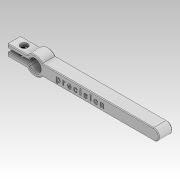
# Autodesk Inventor part: TestLever
Saved by Autodesk Inventor 2020 (Build 240168000, 168)
## iProperties
Created: 2022-01-15
Part Number: TestLever
Material: Generic
Document SubType Name: Modeling
Designer: DDeGo
Density: 1 g/cm^3
Appearance: Default
Author: DDeGo
Autodesk Inventor part; units mm, degrees
ref_plane "YZ Plane" through (0, 0, 0) normal (1, 0, 0) x (0, 1, 0)
ref_plane "XZ Plane" through (0, 0, 0) normal (0, 1, 0) x (-1, 0, 0)
ref_plane "XY Plane" through (0, 0, 0) normal (0, 0, 1) x (1, 0, 0)
sketch "Sketch1" plane through (0, 0, 0) normal (0, 0, 1) x (1, 0, 0)
  line L0 (-32.5361, 0) -> (32.5361, 0) construction
  line L1 (-32.5361, -2.5) -> (32.5361, -2.5)
  line L2 (32.5361, 2.5) -> (-32.5361, 2.5)
  arc A0 (-32.5361, 2.5) -> (-32.5361, -2.5) centre (-32.5361, 0) ccw construction
  arc A1 (32.5361, -2.5) -> (32.5361, 2.5) centre (32.5361, 0) ccw
  circle A2 centre (-20.4639, 0) radius 2.65
  arc A3 (-24.5361, -0.8) -> (-24.5361, 0.8) centre (-20.4639, 0) ccw
  line L3 (-32.5361, 2.5) -> (-32.5361, 0.8)
  line L4 (-32.5361, 0.8) -> (-24.5361, 0.8)
  line L5 (-32.5361, -2.5) -> (-32.5361, -0.8)
  line L6 (-32.5361, -0.8) -> (-24.5361, -0.8)
  line L7 (-24.5361, 0.8) -> (-22.9903, 0.8)
  line L8 (-24.5361, -0.8) -> (-22.9903, -0.8)
  point P0 (0, 0)
  point P1 (-17.1514, 2.5)
  point P2 (-23.7764, 2.5)
  point P3 (-23.7764, -2.5)
  point P4 (-17.1514, -2.5)
  dimension "d0" = 5
  dimension "d2" = 1.7
  dimension "d3" = 8
  dimension "d4" = 5.3
  dimension "d5" = 1.5
  dimension "d11" = 1.6
  dimension "d24" = 53
  constraints: 20 end point, 8 point on circle, 4 centre point, 4 tangent, 3 point on line, 2 parallel, 2 perpendicular, 1 coincident, 1 collinear, 1 horizontal, 1 midpoint, 1 vertical
  measures "d0" distance between parallel lines of L1 L2
  measures "d2" distance of L2.end L3.end
  measures "d3" distance of L3.end L4.end
  measures "d4" diameter of A2
  measures "d5" radial gap between concentric circles of A2 A3
  measures "d11" distance between parallel lines of L6 L4
  measures "d24" distance of L0.end A2.centre
extrude "Extrusion1" add sketch "Sketch1" along normal mid plane 6 contours L5 L6 A3 L1 | A3 L8 A2 L1 | L1 A2 A3 | A3 L2 A1 L1 | L1 A2 L2 A3 | L2 A2 A3 | L7 A3 L2 A2 | A3 L4 L3 L2
sketch "Sketch2" plane through (-32.5361, 2.5, -3) normal (0, 1, 0) x (1, 0, 0)
  line L0 (0, 0) -> (0, -6) construction
  line L1 (8.7597, 0) -> (8.7597, -6) construction
  line L2 (0, 0) -> (8.7597, -6) construction
  circle A0 centre (4.3798, -3) radius 1.6
  point P0 (32.5361, -3)
  dimension "d8" = 3.2
  constraints: 2 end point, 1 centre point, 1 midpoint
  measures "d8" diameter of A0
extrude "Extrusion2" cut sketch "Sketch2" against normal through all
sketch "Sketch3" plane through (0, 0, 0) normal (0, 0, 1) x (1, 0, 0)
  arc A0 (-22.9903, -0.8) -> (-22.9903, 0.8) centre (-20.4639, 0) ccw construction
  line L0 (-17.1514, -2.5) -> (32.5361, -2.5) construction
  line L1 (31.804, -2.5) -> (30.5361, -3.2321)
  line L2 (28.5361, -3.2321) -> (27.2681, -2.5)
  line L3 (31.804, -2.5) -> (27.2681, -2.5)
  arc A1 (28.5361, -3.2321) -> (30.5361, -3.2321) centre (29.5361, -1.5) ccw
  line L4 (29.5361, -3.5) -> (29.5361, -2.5)
  line L5 (-20.4639, 0) -> (-20.4639, -10.7563) construction
  point P0 (0, 0)
  dimension "d12" = 30
  dimension "d13" = 30
  dimension "d14" = 2
  dimension "d15" = 1
  dimension "d16" = 50
  constraints: 10 end point, 3 point on circle, 2 point on line, 2 tangent, 1 centre point, 1 collinear, 1 midpoint, 1 vertical
  measures "d12" angle of L0 L2
  measures "d13" angle of L0 L1
  measures "d14" radius of A1
  measures "d15" distance of L4.start L4.end
  measures "d16" distance from line of L5 L4.start
revolve "Revolution1" add sketch "Sketch3" angle 360 about axis through (29.5361, -3.5, 0) along (0, 1, 0) contours L1 A1 L4 L3
sketch "Sketch4" plane through (0, 0, 3) normal (0, 0, 1) x (1, 0, 0)
  line L0 (-10.945, 1.4249) -> (14.5382, 1.4249) construction
  line L1 (14.5382, 1.4249) -> (14.5382, -2.6227) construction
  line L2 (14.5382, -2.6227) -> (-10.945, -2.6227) construction
  line L3 (-10.945, -2.6227) -> (-10.945, 1.4249) construction
  spline S0 degree 2 poles (-9.0818, -0.2569) (-9.0818, -0.6856) (-9.4734, -1.2029) (-9.8032, -1.2029) knots 0 0 0 1 2 2 2
  spline S1 degree 2 poles (-9.8032, -1.2029) (-10.0855, -1.2029) (-10.2587, -1.0071) knots 0 0 0 1 1 1
  line L4 (-10.2587, -1.0071) -> (-10.2587, -1.883)
  line L5 (-10.2587, -1.883) -> (-10.7554, -1.883)
  line L6 (-10.7554, -1.883) -> (-10.7554, 0.6891)
  line L7 (-10.7554, 0.6891) -> (-10.2958, 0.6891)
  line L8 (-10.2958, 0.6891) -> (-10.2772, 0.5078)
  spline S2 degree 2 poles (-10.2772, 0.5078) (-10.0979, 0.7242) (-9.8073, 0.7242) knots 0 0 0 1 1 1
  spline S3 degree 2 poles (-9.8073, 0.7242) (-9.4631, 0.7242) (-9.0818, 0.2151) (-9.0818, -0.2301) knots 0 0 0 1 2 2 2
  line L9 (-9.0818, -0.2301) -> (-9.0818, -0.2569)
  spline S4 degree 2 poles (-9.5785, -0.2198) (-9.5785, 0.0379) (-9.762, 0.3202) (-9.9371, 0.3202) knots 0 0 0 1 2 2 2
  spline S5 degree 2 poles (-9.9371, 0.3202) (-10.1721, 0.3202) (-10.2587, 0.1409) knots 0 0 0 1 1 1
  line L10 (-10.2587, 0.1409) -> (-10.2587, -0.6196)
  spline S6 degree 2 poles (-10.2587, -0.6196) (-10.168, -0.803) (-9.9351, -0.803) knots 0 0 0 1 1 1
  spline S7 degree 2 poles (-9.9351, -0.803) (-9.5785, -0.803) (-9.5785, -0.2198) knots 0 0 0 1 1 1
  spline S8 degree 2 poles (-6.8559, 0.2233) (-6.9569, 0.2378) (-7.0352, 0.2378) knots 0 0 0 1 1 1
  spline S9 degree 2 poles (-7.0352, 0.2378) (-7.3155, 0.2378) (-7.4042, 0.0482) knots 0 0 0 1 1 1
  line L11 (-7.4042, 0.0482) -> (-7.4042, -1.1678)
  line L12 (-7.4042, -1.1678) -> (-7.9009, -1.1678)
  line L13 (-7.9009, -1.1678) -> (-7.9009, 0.6891)
  line L14 (-7.9009, 0.6891) -> (-7.431, 0.6891)
  line L15 (-7.431, 0.6891) -> (-7.4186, 0.4686)
  spline S10 degree 2 poles (-7.4186, 0.4686) (-7.2681, 0.7242) (-7.0043, 0.7242) knots 0 0 0 1 1 1
  spline S11 degree 2 poles (-7.0043, 0.7242) (-6.9219, 0.7242) (-6.8498, 0.7015) knots 0 0 0 1 1 1
  line L16 (-6.8498, 0.7015) -> (-6.8559, 0.2233)
  spline S12 degree 2 poles (-4.8877, -1.2029) (-5.2958, -1.2029) (-5.809, -0.702) (-5.809, -0.2837) knots 0 0 0 1 2 2 2
  line L17 (-5.809, -0.2837) -> (-5.809, -0.2363)
  spline S13 degree 2 poles (-5.809, -0.2363) (-5.809, 0.044) (-5.5925, 0.4851) (-5.1968, 0.7242) (-4.9413, 0.7242) knots 0 0 0 1 2 3 3 3
  spline S14 degree 2 poles (-4.9413, 0.7242) (-4.56, 0.7242) (-4.123, 0.244) (-4.123, -0.1992) knots 0 0 0 1 2 2 2
  line L18 (-4.123, -0.1992) -> (-4.123, -0.4011)
  line L19 (-4.123, -0.4011) -> (-5.3061, -0.4011)
  spline S15 degree 2 poles (-5.3061, -0.4011) (-5.2813, -0.5825) (-5.0402, -0.803) (-4.8547, -0.803) knots 0 0 0 1 2 2 2
  spline S16 degree 2 poles (-4.8547, -0.803) (-4.5682, -0.803) (-4.4075, -0.5949) knots 0 0 0 1 1 1
  line L20 (-4.4075, -0.5949) -> (-4.1622, -0.869)
  spline S17 degree 2 poles (-4.1622, -0.869) (-4.2735, -1.0256) (-4.6548, -1.2029) (-4.8877, -1.2029) knots 0 0 0 1 2 2 2
  spline S18 degree 2 poles (-4.9433, 0.3243) (-5.0917, 0.3243) (-5.2751, 0.1244) (-5.3019, -0.0631) knots 0 0 0 1 2 2 2
  line L21 (-5.3019, -0.0631) -> (-4.6115, -0.0631)
  line L22 (-4.6115, -0.0631) -> (-4.6115, -0.024)
  spline S19 degree 2 poles (-4.6115, -0.024) (-4.6136, 0.143) (-4.7867, 0.3243) (-4.9433, 0.3243) knots 0 0 0 1 2 2 2
  spline S20 degree 2 poles (-2.1939, -0.803) (-2.0559, -0.803) (-1.8848, -0.6526) (-1.8807, -0.5269) knots 0 0 0 1 2 2 2
  line L23 (-1.8807, -0.5269) -> (-1.4149, -0.5269)
  spline S21 degree 2 poles (-1.4149, -0.5269) (-1.4169, -0.7144) (-1.6189, -1.0297) (-1.9714, -1.2029) (-2.1836, -1.2029) knots 0 0 0 1 2 3 3 3
  spline S22 degree 2 poles (-2.1836, -1.2029) (-2.5835, -1.2029) (-3.0431, -0.6959) (-3.0431, -0.2486) knots 0 0 0 1 2 2 2
  line L24 (-3.0431, -0.2486) -> (-3.0431, -0.2177)
  spline S23 degree 2 poles (-3.0431, -0.2177) (-3.0431, 0.213) (-2.5855, 0.7242) (-2.1878, 0.7242) knots 0 0 0 1 2 2 2
  spline S24 degree 2 poles (-2.1878, 0.7242) (-1.8395, 0.7242) (-1.419, 0.3285) (-1.4149, -0.0013) knots 0 0 0 1 2 2 2
  line L25 (-1.4149, -0.0013) -> (-1.8807, -0.0013)
  spline S25 degree 2 poles (-1.8807, -0.0013) (-1.8848, 0.143) (-2.0559, 0.3243) (-2.196, 0.3243) knots 0 0 0 1 2 2 2
  spline S26 degree 2 poles (-2.196, 0.3243) (-2.3691, 0.3243) (-2.5464, 0.0708) (-2.5464, -0.2136) knots 0 0 0 1 2 2 2
  line L26 (-2.5464, -0.2136) -> (-2.5464, -0.2651)
  spline S27 degree 2 poles (-2.5464, -0.2651) (-2.5464, -0.5516) (-2.3712, -0.803) (-2.1939, -0.803) knots 0 0 0 1 2 2 2
  line L27 (0.2669, -1.1678) -> (-0.2298, -1.1678)
  line L28 (-0.2298, -1.1678) -> (-0.2298, 0.6891)
  line L29 (-0.2298, 0.6891) -> (0.2669, 0.6891)
  line L30 (0.2669, 0.6891) -> (0.2669, -1.1678)
  spline S28 degree 2 poles (-0.2587, 1.1693) (-0.2587, 1.2806) (-0.1103, 1.4249) (0.0196, 1.4249) knots 0 0 0 1 2 2 2
  spline S29 degree 2 poles (0.0196, 1.4249) (0.1453, 1.4249) (0.2978, 1.2806) (0.2978, 1.1693) knots 0 0 0 1 2 2 2
  spline S30 degree 2 poles (0.2978, 1.1693) (0.2978, 1.056) (0.1432, 0.9117) (-0.1061, 0.9117) (-0.2587, 1.056) (-0.2587, 1.1693) knots 0 0 0 1 2 3 4 4 4
  spline S31 degree 2 poles (2.5587, -0.6546) (2.5587, -0.564) (2.3774, -0.4588) (2.1774, -0.4176) knots 0 0 0 1 2 2 2
  spline S32 degree 2 poles (2.1774, -0.4176) (1.5159, -0.2795) (1.5159, 0.145) knots 0 0 0 1 1 1
  spline S33 degree 2 poles (1.5159, 0.145) (1.5159, 0.3923) (1.926, 0.7242) (2.2578, 0.7242) knots 0 0 0 1 2 2 2
  spline S34 degree 2 poles (2.2578, 0.7242) (2.6103, 0.7242) (3.0348, 0.3903) (3.0348, 0.1244) knots 0 0 0 1 2 2 2
  line L31 (3.0348, 0.1244) -> (2.5381, 0.1244)
  spline S35 degree 2 poles (2.5381, 0.1244) (2.5381, 0.2316) (2.4021, 0.3697) (2.2558, 0.3697) knots 0 0 0 1 2 2 2
  spline S36 degree 2 poles (2.2558, 0.3697) (2.13, 0.3697) (1.992, 0.2563) (1.992, 0.1698) knots 0 0 0 1 2 2 2
  spline S37 degree 2 poles (1.992, 0.1698) (1.992, 0.0873) (2.1486, -0.0137) (2.5196, -0.0879) (2.6474, -0.1353) knots 0 0 0 1 2 3 3 3
  spline S38 degree 2 poles (2.6474, -0.1353) (3.041, -0.2795) (3.041, -0.634) knots 0 0 0 1 1 1
  spline S39 degree 2 poles (3.041, -0.634) (3.041, -0.8896) (2.6041, -1.2029) (2.2599, -1.2029) knots 0 0 0 1 2 2 2
  spline S40 degree 2 poles (2.2599, -1.2029) (2.0249, -1.2029) (1.6643, -1.0359) (1.4582, -0.7453) (1.4582, -0.5784) knots 0 0 0 1 2 3 3 3
  line L32 (1.4582, -0.5784) -> (1.9281, -0.5784)
  spline S41 degree 2 poles (1.9281, -0.5784) (1.9342, -0.7103) (2.1156, -0.8504) (2.2702, -0.8504) knots 0 0 0 1 2 2 2
  spline S42 degree 2 poles (2.2702, -0.8504) (2.4124, -0.8504) (2.5587, -0.7433) (2.5587, -0.6546) knots 0 0 0 1 2 2 2
  line L33 (4.7578, -1.1678) -> (4.2611, -1.1678)
  line L34 (4.2611, -1.1678) -> (4.2611, 0.6891)
  line L35 (4.2611, 0.6891) -> (4.7578, 0.6891)
  line L36 (4.7578, 0.6891) -> (4.7578, -1.1678)
  spline S43 degree 2 poles (4.2323, 1.1693) (4.2323, 1.2806) (4.3807, 1.4249) (4.5105, 1.4249) knots 0 0 0 1 2 2 2
  spline S44 degree 2 poles (4.5105, 1.4249) (4.6362, 1.4249) (4.7887, 1.2806) (4.7887, 1.1693) knots 0 0 0 1 2 2 2
  spline S45 degree 2 poles (4.7887, 1.1693) (4.7887, 1.056) (4.6342, 0.9117) (4.3848, 0.9117) (4.2323, 1.056) (4.2323, 1.1693) knots 0 0 0 1 2 3 4 4 4
  spline S46 degree 2 poles (5.9656, -0.2218) (5.9656, 0.0543) (6.1779, 0.4872) (6.5798, 0.7242) (6.8436, 0.7242) knots 0 0 0 1 2 3 3 3
  spline S47 degree 2 poles (6.8436, 0.7242) (7.2187, 0.7242) (7.6948, 0.2646) (7.7216, -0.1311) knots 0 0 0 1 2 2 2
  line L37 (7.7216, -0.1311) -> (7.7257, -0.2589)
  spline S48 degree 2 poles (7.7257, -0.2589) (7.7257, -0.6856) (7.2475, -1.2029) (6.4458, -1.2029) (5.9656, -0.6876) (5.9656, -0.2445) knots 0 0 0 1 2 3 4 4 4
  line L38 (5.9656, -0.2445) -> (5.9656, -0.2218)
  spline S49 degree 2 poles (6.4623, -0.2569) (6.4623, -0.5227) (6.6622, -0.803) (6.8477, -0.803) knots 0 0 0 1 2 2 2
  spline S50 degree 2 poles (6.8477, -0.803) (7.027, -0.803) (7.229, -0.5269) (7.229, -0.2218) knots 0 0 0 1 2 2 2
  spline S51 degree 2 poles (7.229, -0.2218) (7.229, 0.0379) (7.027, 0.3243) (6.8436, 0.3243) knots 0 0 0 1 2 2 2
  spline S52 degree 2 poles (6.8436, 0.3243) (6.6622, 0.3243) (6.4623, 0.0399) (6.4623, -0.2569) knots 0 0 0 1 2 2 2
  line L39 (9.3642, 0.6891) -> (9.3786, 0.4748)
  spline S53 degree 2 poles (9.3786, 0.4748) (9.5785, 0.7242) (9.9124, 0.7242) knots 0 0 0 1 1 1
  spline S54 degree 2 poles (9.9124, 0.7242) (10.2092, 0.7242) (10.4977, 0.3779) (10.4998, 0.0317) knots 0 0 0 1 2 2 2
  line L40 (10.4998, 0.0317) -> (10.4998, -1.1678)
  line L41 (10.4998, -1.1678) -> (10.0051, -1.1678)
  line L42 (10.0051, -1.1678) -> (10.0051, 0.0193)
  spline S55 degree 2 poles (10.0051, 0.0193) (10.0051, 0.178) (9.8671, 0.3202) (9.7063, 0.3202) knots 0 0 0 1 2 2 2
  spline S56 degree 2 poles (9.7063, 0.3202) (9.4981, 0.3202) (9.393, 0.1409) knots 0 0 0 1 1 1
  line L43 (9.393, 0.1409) -> (9.393, -1.1678)
  line L44 (9.393, -1.1678) -> (8.8963, -1.1678)
  line L45 (8.8963, -1.1678) -> (8.8963, 0.6891)
  line L46 (8.8963, 0.6891) -> (9.3642, 0.6891)
  point P0 (0, 0)
  constraints: 2 other
extrude "Extrusion3" cut sketch "Sketch4" against normal blind 0.2
fillet "Fillet1" radius 1 2 edges at (-22.9903, -0.8, 0) (-22.9903, 0.8, 0)
chamfer "Chamfer1" distance 0.3 angle 45 28 edges at (7.6923, 2.5, -3) (35.0361, 0, -3) (7.6923, -2.5, -3) (-20.4639, 4.15, -3) (-28.1562, 2.5, -3) (-20.4639, -4.15, -3) (-28.1562, -2.5, -3) (-32.5361, -1.65, -3) (-32.5361, 1.65, -3) (-17.8139, 0, -3) (-23.1358, 0.936, -3) (-28.0876, 0.8, -3) (-23.1358, -0.936, -3) (-28.0876, -0.8, -3) (-17.8139, 0, 3) (-23.1358, -0.936, 3) (-28.0876, -0.8, 3) (-23.1358, 0.936, 3) (-28.0876, 0.8, 3) (-28.1562, 2.5, 3) (-32.5361, 1.65, 3) (-32.5361, -1.65, 3) (-28.1562, -2.5, 3) (-20.4639, 4.15, 3) (7.6923, 2.5, 3) (35.0361, 0, 3) (7.6923, -2.5, 3) (-20.4639, -4.15, 3)
body "Solid1"
